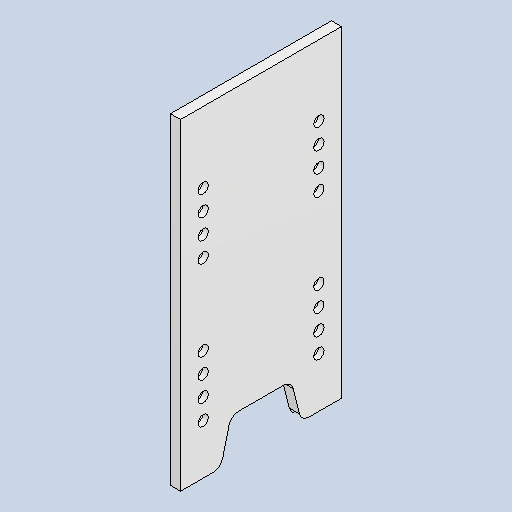
# Autodesk Inventor part: Ramp
Saved by Autodesk Inventor 2023.2 (Build 272271000, 271)
## iProperties
Created: 2024-02-17
Part Number: Ramp
Material: UHMW, White
Document SubType Name: Modeling
Designer: Nathan Cai
Density: 0.94 g/cm^3
Appearance: Smooth - White
Mass: 12.0698 g
Surface Area: 95.7512 cm^2
Volume: 12.8403 cm^3
Author: Nathan Cai
Autodesk Inventor part; units mm, degrees
ref_plane "YZ Plane" through (0, 0, 0) normal (1, 0, 0) x (0, 1, 0)
ref_plane "XZ Plane" through (0, 0, 0) normal (0, 1, 0) x (-1, 0, 0)
ref_plane "XY Plane" through (0, 0, 0) normal (0, 0, 1) x (1, 0, 0)
sketch "Sketch1" plane through (0, 0, 0) normal (1, 0, 0) x (0, 1, 0)
  line L0 (50.8, 25.4) -> (-50.8, 25.4)
  line L1 (-50.8, 25.4) -> (-50.8, -25.4)
  line L2 (-50.8, -25.4) -> (50.8, -25.4)
  line L3 (50.8, -25.4) -> (50.8, 25.4)
  line L4 (50.8, 25.4) -> (-50.8, -25.4) construction
  line L5 (-50.8, 25.4) -> (50.8, -25.4) construction
  line L6 (0, 0) -> (-50.8, 0) construction
  line L7 (-38.1, -9.525) -> (-50.8, -9.525)
  line L8 (-50.8, -9.525) -> (-50.8, 9.525)
  line L9 (-50.8, 9.525) -> (-38.1, 9.525)
  line L10 (-38.1, 9.525) -> (-38.1, -9.525)
  line L11 (-38.1, -9.525) -> (-50.8, 9.525) construction
  line L12 (-50.8, -9.525) -> (-38.1, 9.525) construction
  line L13 (-38.1, -9.525) -> (-50.8, -12.7)
  line L14 (-38.1, 9.525) -> (-50.8, 12.7)
  line L15 (0, -25.4) -> (0, 25.4) construction
  line L16 (38.1, -9.525) -> (50.8, -9.525) construction
  line L17 (50.8, -9.525) -> (50.8, 9.525)
  line L18 (50.8, 9.525) -> (38.1, 9.525) construction
  line L19 (38.1, 9.525) -> (38.1, -9.525)
  line L20 (38.1, -9.525) -> (50.8, 9.525) construction
  line L21 (50.8, -9.525) -> (38.1, 9.525) construction
  line L22 (38.1, -9.525) -> (50.8, -12.7)
  line L23 (38.1, 9.525) -> (50.8, 12.7)
  point P0 (-44.45, 0)
  point P1 (50.8, 0)
  point P2 (44.45, 0)
  point P3 (50.8, -12.7)
  dimension "d0" = 101.6
  dimension "d1" = 50.8
  dimension "d19" = 12.7
  dimension "d20" = 19.05
  dimension "d21" = 12.7
  constraints: 48 end point, 9 symmetric about line, 7 midpoint, 4 parallel, 3 point on line, 2 horizontal, 2 perpendicular
  measures "d0" distance of L2.end L1.end
  measures "d1" distance of L1.end L0.end
  measures "d19" distance of L8.end L9.end
  measures "d20" distance of L7.end L8.end
  measures "d21" distance from line of L2 L13.end
extrude "Extrusion1" add sketch "Sketch1" along normal blind 3.175 contours L3 L23 L19 L22 L2 L1 L13 L10 L14 L0 | L3 L22 L19 L23
fillet "Fillet2" radius 3.175 4 edges at (1.5875, -38.1, 9.525) (1.5875, -50.8, 12.7) (1.5875, -38.1, -9.525) (1.5875, -50.8, -12.7)
sketch "Sketch5" plane through (0, 0, 0) normal (-1, 0, 0) x (0, 0, 1)
  point P0 (18.2563, -35.0209)
  point P1 (18.2563, -28.6709)
  point P2 (18.2563, -22.3209)
  point P3 (18.2563, -15.9709)
  point P4 (18.2563, 9.4291)
  point P5 (18.2563, 15.7791)
  point P6 (18.2563, 22.1291)
  point P7 (18.2563, 28.4791)
  point P8 (-18.2562, 28.4791)
  point P9 (-18.2562, 22.1291)
  point P10 (-18.2562, 15.7791)
  point P11 (-18.2562, 9.4291)
  point P12 (-18.2562, -15.9709)
  point P13 (-18.2562, -22.3209)
  point P14 (-18.2562, -28.6709)
  point P15 (-18.2562, -35.0209)
hole "Hole3" at (0, -35.0209, 18.2563) at (0, -28.6709, 18.2563) at (0, -22.3209, 18.2563) at (0, -15.9709, 18.2563) at (0, 9.4291, 18.2563) at (0, 15.7791, 18.2563) at (0, 22.1291, 18.2563) at (0, 28.4791, 18.2563) at (0, 28.4791, -18.2562) at (0, 22.1291, -18.2562) at (0, 15.7791, -18.2562) at (0, 9.4291, -18.2562) at (0, -15.9709, -18.2562) at (0, -22.3209, -18.2562) at (0, -28.6709, -18.2562) at (0, -35.0209, -18.2562) direction (1, 0, 0) diameter 3.2639 end through all countersink diameter 5.715 countersink angle 82
body "Solid1"
